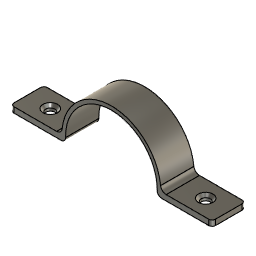
cable-bracket (Autodesk Fusion 360 design; units mm, degrees)
Autodesk Fusion 360 part; units mm, degrees
sketch "Sketch1" plane through (0, 0, 0) normal (0, 0, 1) x (1, 0, 0)
sketch "Sketch2" plane through (0, 0, 0) normal (0, 1, 0) x (1, 0, 0)
  circle A0 centre (0, 0) radius 25
  circle A1 centre (0, 0) radius 27
  line L0 (-55, 0) -> (55, 0)
  line L1 (-55, 0) -> (-55, 3)
  line L2 (-55, 3) -> (55, 3)
  line L3 (55, 0) -> (55, 3)
  dimension "d1" = 50
  dimension "d2" = 2
  constraint coincident A0.centre A1.centre
  constraint horizontal L0
  constraint perpendicular L0 L1
  constraint perpendicular L1 L2
  constraint perpendicular L0 L3
  measures "d1" diameter of A0
extrude "Extrude1" add sketch "Sketch2" along normal blind 18.166 contours A0 A1 L0 | A0 A1 L0 L2 | A0 A1 L0 L2 | A1 L0 L2 L3 | A1 L0 L1 L2
fillet "Fillet1" radius 3.06 2 edges at (-27, 9.083, 0) (27, 9.083, 0)
fillet "Fillet2" radius 2.455 2 edges at (-24.8193, 9.083, -3) (24.8193, 9.083, -3)
fillet "Fillet3" radius 1.852 4 edges at (-55, 0, -1.5) (-55, 18.166, -1.5) (55, 0, -1.5) (55, 18.166, -1.5)
hole "Hole1" at (42.4144, 9.083, 0) direction (0, 0, -1) diameter 5 depth 7 tip angle 118 countersink diameter 8 countersink angle 90
hole "Hole2" at (-42.4144, 9.083, 0) direction (0, 0, -1) diameter 5 depth 7 tip angle 118 countersink diameter 8 countersink angle 90
